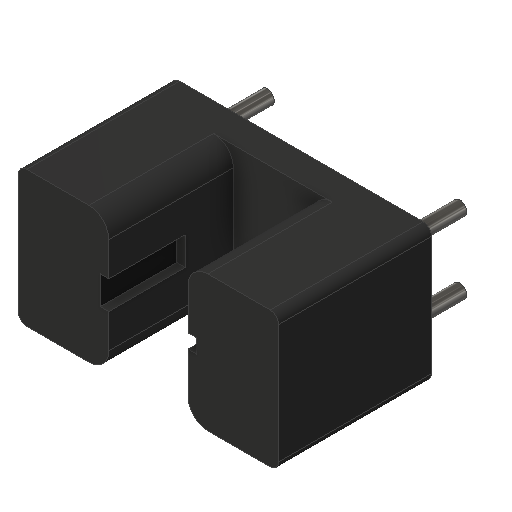
# Autodesk Inventor part: COTS_Vishay_TCST1230_Optocoupler
Saved by Autodesk Inventor 2026.1 (Build 301233000, 233)
## iProperties
Created: 2018-07-20
Part Number: COTS_Vishay_TCST1230_Optocoupler
Material: ABS Plastic
Document SubType Name: Modeling
Designer: Andrzej
Density: 1.06 g/cm^3
Appearance: Rubber - Black
Author: Andrzej
Autodesk Inventor part; units mm, degrees
ref_plane "YZ Plane" through (0, 0, 0) normal (1, 0, 0) x (0, 1, 0)
ref_plane "XZ Plane" through (0, 0, 0) normal (0, 1, 0) x (-1, 0, 0)
ref_plane "XY Plane" through (0, 0, 0) normal (0, 0, 1) x (1, 0, 0)
sketch "Sketch1" plane through (0, 0, 0) normal (0, 0, 1) x (1, 0, 0)
  line L0 (-4.3779, 2.8981) -> (4.8221, 2.8981)
  line L1 (4.8221, 2.8981) -> (4.8221, -1.9019)
  line L2 (4.8221, -1.9019) -> (-4.3779, -1.9019)
  line L3 (-4.3779, -1.9019) -> (-4.3779, 2.8981)
  line L4 (-1.1779, 2.8981) -> (-1.1779, -1.9019)
  line L5 (1.6221, 2.8981) -> (1.6221, -1.9019)
  point P0 (0, 0)
  dimension "d0" = 2.8
  dimension "d1" = 9.2
  dimension "d2" = 3.2
  dimension "d11" = 4.8
  constraints: 12 end point, 4 point on line, 3 parallel, 2 perpendicular, 1 horizontal
  measures "d0" distance between parallel lines of L5 L4
  measures "d1" distance between parallel lines of L1 L3
  measures "d2" distance between parallel lines of L3 L4
  measures "d11" distance of L0.end L1.end
extrude "Extrusion1" add sketch "Sketch1" along normal blind 4.4 contours L0 L4 L2 L3 | L0 L1 L2 L5
extrude "Extrusion2" add sketch "Sketch1" against normal blind 1
sketch "Sketch2" plane through (0, 0, -1) normal (0, 0, -1) x (-1, 0, 0)
  line L0 (4.3779, 2.8981) -> (-4.8221, 2.8981) projected
  line L1 (-4.8221, 2.8981) -> (-4.8221, -1.9019) projected
  line L2 (-4.8221, -1.9019) -> (4.3779, -1.9019) projected
  line L3 (4.3779, -1.9019) -> (4.3779, 2.8981) projected
  circle A0 centre (-3.6221, 1.7681) radius 0.25
  circle A1 centre (-3.6221, -0.7719) radius 0.25
  circle A2 centre (3.1779, 1.7681) radius 0.25
  circle A3 centre (3.1779, -0.7719) radius 0.25
  point P0 (0, 0)
  dimension "d7" = 2.54
  dimension "d8" = 6.8
  dimension "d9" = 9.2
  dimension "d10" = 4.8
  dimension "d12" = 1.13
  dimension "d13" = 1.2
  dimension "d14" = 0.5
  dimension "d15" = 0.5
  dimension "d16" = 0.5
  dimension "d17" = 0.5
  constraints: 4 centre point, 4 coincident, 2 horizontal alignment, 2 vertical alignment
  measures "d7" distance of point (-3.622, -0.772) point (-3.622, 1.768)
  measures "d8" distance of point (3.178, 1.768) point (-3.622, 1.768)
  measures "d9" distance of L1.end L2.end
  measures "d10" distance of L0.end L1.end
  measures "d12" distance from line of point (-3.622, 1.768) L0
  measures "d13" distance from line of L1 point (-3.622, 1.768)
  measures "d14" diameter of A0
  measures "d15" diameter of A1
  measures "d16" diameter of A2
  measures "d17" diameter of A3
extrude "Extrusion3" add sketch "Sketch2" along normal blind 2.2 contours A0 | A1 | A2 | A3
sketch "Sketch3" plane through (0, 0, 4.4) normal (0, 0, 1) x (1, 0, 0)
  line L0 (4.8221, -1.9019) -> (4.8221, 2.8981) projected
  line L1 (4.8221, 2.8981) -> (1.6221, 2.8981) projected
  line L2 (1.6221, 2.8981) -> (1.6221, -1.9019) projected
  line L3 (1.6221, -1.9019) -> (4.8221, -1.9019) projected
  line L4 (-4.3779, 2.8981) -> (-4.3779, -1.9019) projected
  line L5 (-4.3779, -1.9019) -> (-1.1779, -1.9019) projected
  line L6 (-1.1779, -1.9019) -> (-1.1779, 2.8981) projected
  line L7 (-1.1779, 2.8981) -> (-4.3779, 2.8981) projected
  line L8 (1.6221, 2.8981) -> (1.6221, -1.9019) projected
  line L9 (1.6221, 0.2481) -> (1.9221, 0.2481)
  line L10 (1.9221, 0.2481) -> (1.9221, 0.7481)
  line L11 (1.9221, 0.7481) -> (1.6221, 0.7481)
  line L12 (1.6221, 0.7481) -> (1.6221, 0.2481)
  line L13 (-1.1779, -0.0019) -> (-1.4779, -0.0019)
  line L14 (-1.4779, -0.0019) -> (-1.4779, 0.9981)
  line L15 (-1.4779, 0.9981) -> (-1.1779, 0.9981)
  line L16 (-1.1779, 0.9981) -> (-1.1779, -0.0019)
  point P0 (0, 0)
  dimension "d20" = 0.3
  dimension "d21" = 0.5
  dimension "d22" = 0.3
  dimension "d23" = 1
  dimension "d24" = 4.8
  dimension "d25" = 2.15
  dimension "d26" = 1.9
  constraints: 16 end point, 4 parallel, 2 horizontal, 2 perpendicular, 2 point on line
  measures "d20" distance of L11.end L10.end
  measures "d21" distance of L10.end L9.end
  measures "d22" distance of L14.end L15.end
  measures "d23" distance of L13.end L14.end
  measures "d24" distance of L0.start L0.end
  measures "d25" distance between parallel lines of L3 L9
  measures "d26" distance between parallel lines of L5 L13
extrude "Extrusion4" cut sketch "Sketch3" against normal blind 2.7 contours L2 L11 L10 L9 | L6 L13 L14 L15
fillet "Fillet1" radius 0.7 4 edges at (1.6221, -1.9019, 2.2) (1.6221, 2.8981, 2.2) (-1.1779, 2.8981, 2.2) (-1.1779, -1.9019, 2.2)
fillet "Fillet1" radius 0.3 4 edges at (-4.3779, -1.9019, 1.7) (-4.3779, 2.8981, 1.7) (4.8221, 2.8981, 1.7) (4.8221, -1.9019, 1.7)
equation "\"d2\" = -0.5 * d0 + 0.5 * d1"
equation "\"d12\" = -0.5 * d7 + 0.5 * d10"
equation "\"d13\" = -0.5 * d8 + 0.5 * d9"
equation "\"d20\" = d22"
equation "\"d25\" = -0.5 * d21 + 0.5 * d24"
equation "\"d26\" = -0.5 * d23 + 0.5 * d24"
body "Solid1"
